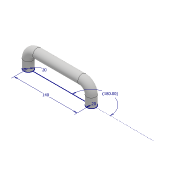
# Autodesk Inventor part: handle_140_20
Saved by Autodesk Inventor 2018 (Build 220112000, 112)
## iProperties
Created: 2018-04-02
Part Number: handle_140_20
Material: Generic
Document SubType Name: Modeling
Designer: Bardo91
Density: 1 g/cm^3
Appearance: Default
Author: Bardo91
Autodesk Inventor part; units mm, degrees
ref_plane "YZ Plane" through (0, 0, 0) normal (1, 0, 0) x (0, 1, 0)
ref_plane "XZ Plane" through (0, 0, 0) normal (0, 1, 0) x (-1, 0, 0)
ref_plane "XY Plane" through (0, 0, 0) normal (0, 0, 1) x (1, 0, 0)
sketch "Sketch1" plane through (0, 0, 0) normal (0, 0, 1) x (1, 0, 0)
  circle A0 centre (0, 0) radius 10
  line L0 (0, 0) -> (-140, 0)
  line L1 (0, 0) -> (140, 0) construction
  circle A1 centre (-140, 0) radius 10
  dimension "d0" = 20
  dimension "d1" = 140
  dimension "d2" = 180
  dimension "d3" = 20
  constraints: 4 end point, 2 centre point, 2 coincident, 2 horizontal, 1 collinear
  measures "d0" diameter of A0
  measures "d1" distance of L0.start L0.end
  measures "d2" angle of L0 L1
  measures "d3" diameter of A1
sketch "Sketch2" plane through (0, 0, 0) normal (0, 1, 0) x (-1, 0, 0)
  line L0 (0, 0) -> (0, 20)
  line L1 (20, 40) -> (120, 40)
  line L2 (140, 20) -> (140, 0)
  arc A0 (140, 20) -> (120, 40) centre (120, 20) ccw
  arc A1 (20, 40) -> (0, 20) centre (20, 20) ccw
  point P0 (0, 40)
  point P1 (140, 40)
  dimension "d4" = 40
  dimension "d5" = 140
  dimension "d6" = 20
  constraints: 6 end point, 4 point on circle, 4 point on line, 4 tangent, 2 centre point, 2 perpendicular, 1 equal radius, 1 vertical
  measures "d4" distance of L0.start point (0, 40)
  measures "d5" distance of point (0, 40) point (140, 40)
  measures "d6" radius of A0
sweep "Sweep1" add profiles "Sketch1" path "Sketch2" path curves L2 A0 L1 A1 contours A1
extrude "Extrusion1" add sketch "Sketch1" along normal up to surface (20 mm away) contours A0
body "Solid1"
